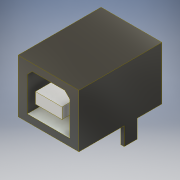
# Autodesk Inventor part: USB-B
Saved by Autodesk Inventor 2016 (Build 200138000, 138)
## iProperties
Created: 2016-09-23
Part Number: USB-B
Material: Generic
Document SubType Name: Modeling
Designer: jfixelle
Density: 1 g/cm^3
Appearance: Silver
Author: jfixelle
Autodesk Inventor part; units mm, degrees
ref_plane "YZ Plane" through (0, 0, 0) normal (1, 0, 0) x (0, 1, 0)
ref_plane "XZ Plane" through (0, 0, 0) normal (0, 1, 0) x (-1, 0, 0)
ref_plane "XY Plane" through (0, 0, 0) normal (0, 0, 1) x (1, 0, 0)
sketch "Sketch1" plane through (0, 0, 0) normal (0, 0, 1) x (1, 0, 0)
  line L0 (-6.05, 10.9) -> (6.05, 10.9)
  line L1 (6.05, 10.9) -> (6.05, 0.3)
  line L2 (6.05, 0.3) -> (-6.05, 0.3)
  line L3 (-6.05, 0.3) -> (-6.05, 10.9)
  point P0 (0, 0)
  dimension "d0" = 10.6
  dimension "d1" = 0.3
  dimension "d2" = 12.1
  dimension "d3" = 6.05
  constraints: 8 end point, 2 parallel, 1 horizontal, 1 perpendicular
  measures "d0" distance of L0.end L1.end
  measures "d1" distance from line of point (0, 0) L2
  measures "d2" distance of L0.start L0.end
  measures "d3" distance from line of point (0, 0) L1
extrude "Extrusion1" add sketch "Sketch1" against normal blind 16.5
sketch "Sketch2" plane through (-6.05, 0.3, 0) normal (0, -1, 0) x (1, 0, 0)
  line L0 (9.4241, -4.8692) -> (1.7869, -4.8692)
  line L1 (1.7869, -4.8692) -> (1.7869, -15.7795)
  line L2 (1.7869, -15.7795) -> (9.4241, -15.7795)
  line L3 (9.4241, -15.7795) -> (9.4241, -4.8692)
  point P0 (6.05, 0)
  constraints: 8 end point, 2 parallel, 1 horizontal, 1 perpendicular
extrude "Extrusion2" add sketch "Sketch2" along normal blind 0.3
sketch "Sketch3" plane through (-6.05, 0, 0) normal (0, -1, 0) x (1, 0, 0)
  circle A0 centre (4.8, -15.01) radius 0.3
  circle A1 centre (7.3, -15.01) radius 0.3
  circle A2 centre (4.8, -13.01) radius 0.3
  circle A3 centre (7.3, -13.01) radius 0.3
  line L0 (12.1, 0) -> (0, 0) projected
  point P0 (6.05, 0)
  dimension "d8" = 1.25
  dimension "d9" = 1.25
  dimension "d10" = 0
  dimension "d11" = 0
  dimension "d12" = 2
  dimension "d13" = 0
  dimension "d14" = 0
  dimension "d15" = 13.01
  dimension "d16" = 0.6
  dimension "d17" = 0.6
  dimension "d18" = 0.6
  dimension "d19" = 0.6
  constraints: 4 centre point
  measures "d8" horizontal distance of point (6.05, 0) A3.centre
  measures "d9" horizontal distance of point (6.05, 0) A2.centre
  measures "d10" horizontal distance of A3.centre A1.centre
  measures "d11" horizontal distance of A0.centre A2.centre
  measures "d12" distance of A3.centre A1.centre
  measures "d13" vertical distance of A3.centre A2.centre
  measures "d14" vertical distance of A1.centre A0.centre
  measures "d15" distance from line of A3.centre L0
  measures "d16" diameter of A1
  measures "d17" diameter of A3
  measures "d18" diameter of A2
  measures "d19" diameter of A0
extrude "Extrusion3" add sketch "Sketch3" along normal blind 2.8
sketch "Sketch4" plane through (-6.05, 0.3, 0) normal (0, -1, 0) x (1, 0, 0)
  line L0 (12.1, 0) -> (12.1, -16.5) projected
  line L1 (12.1, -9) -> (11.4, -9)
  line L2 (11.4, -9) -> (11.4, -11.6)
  line L3 (11.4, -11.6) -> (12.1, -11.6)
  line L4 (12.1, -11.6) -> (12.1, -9)
  line L5 (0, 0) -> (0, -16.5) projected
  line L6 (0, -9) -> (0.7, -9)
  line L7 (0.7, -9) -> (0.7, -11.6)
  line L8 (0.7, -11.6) -> (0, -11.6)
  line L9 (0, -11.6) -> (0, -9)
  line L10 (12.1, 0) -> (0, 0) projected
  point P0 (6.05, 0)
  dimension "d22" = 2.6
  dimension "d23" = 2.6
  dimension "d24" = 9
  dimension "d25" = 0
  dimension "d26" = 0.7
  dimension "d27" = 0.7
  constraints: 16 end point, 4 parallel, 2 horizontal, 2 perpendicular, 2 point on line
  measures "d22" distance of L6.end L7.end
  measures "d23" distance of L1.end L2.end
  measures "d24" distance between parallel lines of L10 L1
  measures "d25" distance between parallel lines of L1 L6
  measures "d26" distance of L1.start L1.end
  measures "d27" distance of L6.start L6.end
extrude "Extrusion4" add sketch "Sketch4" along normal blind 3.6
sketch "Sketch5" plane through (0, 0, 0) normal (0, 0, 1) x (1, 0, 0)
  line L0 (-4.225, 1.71) -> (4.225, 1.71)
  line L1 (4.225, 1.71) -> (4.225, 9.49)
  line L2 (4.225, 9.49) -> (-4.225, 9.49)
  line L3 (-4.225, 9.49) -> (-4.225, 1.71)
  line L4 (6.05, 0.3) -> (-6.05, 0.3) projected
  line L5 (-3.225, 9.49) -> (-4.225, 8.49)
  line L6 (3.225, 9.49) -> (4.225, 8.49)
  point P0 (0, 0)
  dimension "d30" = 7.78
  dimension "d31" = 8.45
  dimension "d32" = 4.225
  dimension "d33" = 1.41
  dimension "d34" = 45
  dimension "d35" = 45
  dimension "d36" = 1
  dimension "d37" = 1
  constraints: 12 end point, 4 point on line, 2 parallel, 1 horizontal, 1 perpendicular
  measures "d30" distance of L0.end L1.end
  measures "d31" distance of L1.end L2.end
  measures "d32" distance from line of point (0, 0) L1
  measures "d33" distance between parallel lines of L4 L0
  measures "d34" angle of L2 L6
  measures "d35" angle of L2 L5
  measures "d36" distance from line of L2 L5.end
  measures "d37" distance from line of L2 L6.end
extrude "Extrusion5" cut sketch "Sketch5" against normal blind 8 contours L3 L5 L2 L6 L1 L0
sketch "Sketch6" plane through (0, 0, -8) normal (0, 0, 1) x (1, 0, 0)
  line L0 (-2.6112, 6.3628) -> (2.6965, 6.3628)
  line L1 (2.6965, 6.3628) -> (2.6965, 4.1886)
  line L2 (2.6965, 4.1886) -> (-2.6112, 4.1886)
  line L3 (-2.6112, 4.1886) -> (-2.6112, 6.3628)
  point P0 (0, 0)
  constraints: 8 end point, 2 parallel, 1 horizontal, 1 perpendicular
extrude "Extrusion6" add sketch "Sketch6" along normal blind 8
body "Solid1"
